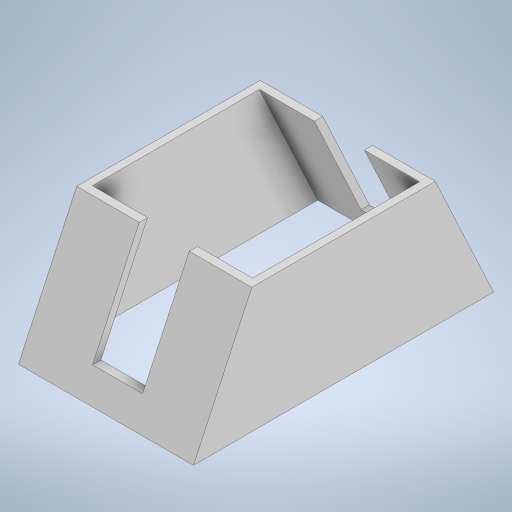
# Autodesk Inventor part: Pie
Saved by Autodesk Inventor 2023 (Build 270158000, 158)
## iProperties
Created: 2022-10-19
Part Number: Pie
Material: Generic
Document SubType Name: Modeling
Designer: User
Density: 1 g/cm^3
Appearance: Default
Author: User
## iProperties of the stored document Pie_3DPrint.ipt
Created: 2022-11-02
Part Number: Pie_3DPrint
Material: Generic
Document SubType Name: Modeling
Designer: diego
Density: 1 g/cm^3
Appearance: Default
Author: diego
Autodesk Inventor part; units mm, degrees
ref_plane "YZ Plane" through (0, 0, 0) normal (1, 0, 0) x (0, 1, 0)
ref_plane "XZ Plane" through (0, 0, 0) normal (0, 1, 0) x (-1, 0, 0)
ref_plane "XY Plane" through (0, 0, 0) normal (0, 0, 1) x (1, 0, 0)
sketch "Sketch1" plane through (0, 0, 0) normal (1, 0, 0) x (0, 1, 0)
  line L0 (0, 0) -> (0, -120)
  line L1 (0, -120) -> (50, -96.6846)
  line L2 (0, 0) -> (50, -23.3154)
  line L3 (50, -23.3154) -> (50, -96.6846)
  dimension "d0" = 120
  dimension "d1" = 65
  dimension "d2" = 65
  dimension "d3" = 50
  dimension "d4" = 50
  constraints: 8 end point, 1 vertical
  measures "d0" distance of L0.start L0.end
  measures "d1" angle of L1 L0
  measures "d2" angle of L2 L0
  measures "d3" horizontal distance of L0.end L1.end
  measures "d4" horizontal distance of L0.start L2.end
extrude "Extrusion1" add sketch "Sketch1" along normal blind 70
shell "Shell1" thickness 3 removed faces 2 at (23.3333, 50, -72.2282) at (23.3333, 0, -40)
sketch "Sketch2" plane through (0, 50, -23.3154) normal (0, 1, 0) x (1, 0, 0)
  line L0 (35, 37.1714) -> (45, 37.1714) construction
  line L1 (35, 37.1714) -> (25, 37.1714) construction
  line L2 (0, 96.6846) -> (70, 96.6846) projected
  line L3 (25, 96.6846) -> (25, -23.3154)
  line L4 (0, -23.3154) -> (70, -23.3154) projected
  line L5 (45, 96.6846) -> (45, -23.3154)
  line L6 (45, -23.3154) -> (25, -23.3154)
  line L7 (25, 96.6846) -> (45, 96.6846)
  point P0 (45, -23.3154)
  dimension "d8" = 10
  dimension "d9" = 10
  dimension "d10" = 20
  constraints: 12 end point, 2 horizontal, 2 point on line, 2 vertical, 1 parallel, 1 perpendicular
  measures "d8" distance of L0.start L0.end
  measures "d9" distance of L0.start L1.end
  measures "d10" distance between parallel lines of L3 L5
extrude "Extrusion2" cut sketch "Sketch2" against normal blind 40
body "Solid1"
